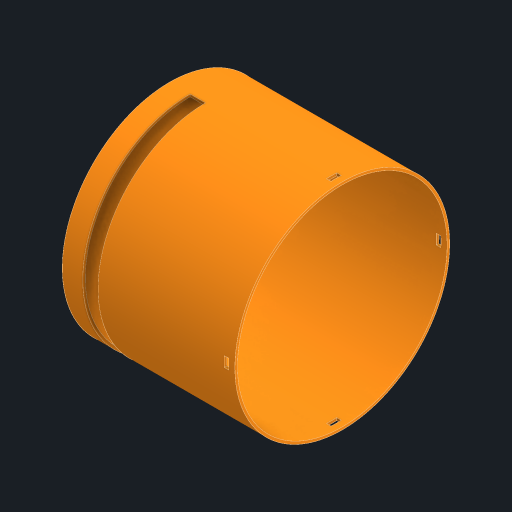
# Autodesk Inventor part: OUTK_001_ChipBucket
Saved by Autodesk Inventor 2024.2 (Build 282272000, 272)
## iProperties
Created: 2024-11-24
Part Number: OUTK_001_ChipBucket
Material: Polyethylene, High Density
Document SubType Name: Modeling
Designer: Bryan
Density: 0.952 g/cm^3
Appearance: Orange
Mass: 1203.08 g
Surface Area: 4862.89 cm^2
Volume: 1263.74 cm^3
Author: Bryan
Autodesk Inventor part; units mm, degrees
ref_plane "YZ Plane" through (0, 0, 0) normal (1, 0, 0) x (0, 1, 0)
ref_plane "XZ Plane" through (0, 0, 0) normal (0, 1, 0) x (-1, 0, 0)
ref_plane "XY Plane" through (0, 0, 0) normal (0, 0, 1) x (1, 0, 0)
sketch "Sketch1" plane through (0, 0, 0) normal (1, 0, 0) x (0, 1, 0)
  circle A0 centre (0, 0) radius 133.35
  dimension "d0" = 266.7
  constraints: 1 centre point, 1 coincident
  measures "d0" diameter of A0
extrude "Extrusion1" add sketch "Sketch1" along normal mid plane 214.3435
sketch "Sketch2" plane through (107.1717, 0, 0) normal (1, 0, 0) x (0, 0, -1)
  circle A0 centre (0, 0) radius 130.175
  dimension "d3" = 260.35
  constraints: 1 centre point, 1 coincident
  measures "d3" diameter of A0
extrude "Extrusion2" cut sketch "Sketch2" against normal blind 201.6435
sketch "Sketch3" plane through (0, 0, 0) normal (0, 0, 1) x (1, 0, 0)
  line L0 (107.1717, 130.175) -> (107.1717, -130.175) projected
  line L1 (107.1717, 130.175) -> (-94.4717, 130.175) projected
  line L2 (107.1717, -130.175) -> (-94.4717, -130.175) projected
  line L3 (-81.7717, 130.175) -> (-81.7717, -130.175)
  line L4 (-62.7217, -130.175) -> (-62.7217, 130.175)
  line L5 (-94.4717, 130.175) -> (-94.4717, -130.175) projected
  point P0 (0, 0)
  point P1 (-139.7, 130.175)
  point P2 (-139.7, -130.175)
  dimension "d7" = 19.05
  dimension "d61" = 12.7
  constraints: 4 end point, 4 point on line, 1 parallel, 1 vertical
  measures "d7" distance between parallel lines of L3 L4
  measures "d61" distance between parallel lines of L3 L5
extrude "Extrusion3" cut sketch "Sketch3" along normal blind 266.7 contours L4 L2 L3 L1
sketch "Sketch4" plane through (0, 0, 0) normal (0, 1, 0) x (-1, 0, 0)
  line L0 (81.7717, 0) -> (62.7217, 0) projected
  line L1 (81.7717, 0) -> (81.7717, 28.9256) projected
  line L2 (62.7217, 0) -> (62.7217, 28.9256) projected
  line L3 (62.7217, 28.9256) -> (81.7717, 28.9256) projected
  point P0 (0, 0)
extrude "Extrusion4" cut sketch "Sketch4" along normal through all both and the other way through all
sketch "Sketch5" plane through (0, 0, 0) normal (0, 1, 0) x (-1, 0, 0)
  line L0 (-93.8367, 6.35) -> (-99.5517, 6.35)
  line L1 (-99.5517, 6.35) -> (-99.5517, -6.35)
  line L2 (-99.5517, -6.35) -> (-93.8367, -6.35)
  line L3 (-93.8367, -6.35) -> (-93.8367, 6.35)
  line L4 (-107.1717, 133.35) -> (-107.1717, -133.35) projected
  point P0 (0, 0)
  point P1 (-93.8367, 0)
  dimension "d12" = 5.715
  dimension "d13" = 12.7
  dimension "d14" = 7.62
  constraints: 8 end point, 2 parallel, 1 horizontal, 1 horizontal alignment, 1 midpoint, 1 perpendicular
  measures "d12" distance of L2.end L1.end
  measures "d13" distance of L1.end L0.end
  measures "d14" distance between parallel lines of L4 L1
extrude "Extrusion5" cut sketch "Sketch5" along normal through all both and the other way through all
sketch "Sketch6" plane through (0, 0, 0) normal (0, 0, 1) x (1, 0, 0)
  line L0 (93.8367, 6.35) -> (99.5517, 6.35)
  line L1 (99.5517, 6.35) -> (99.5517, -6.35)
  line L2 (99.5517, -6.35) -> (93.8367, -6.35)
  line L3 (93.8367, -6.35) -> (93.8367, 6.35)
  line L4 (107.1717, -133.35) -> (107.1717, 133.35) projected
  point P0 (0, 0)
  point P1 (93.8367, 0)
  dimension "d17" = 5.715
  dimension "d18" = 12.7
  dimension "d19" = 7.62
  constraints: 8 end point, 2 parallel, 1 horizontal, 1 horizontal alignment, 1 midpoint, 1 perpendicular
  measures "d17" distance of L1.end L2.end
  measures "d18" distance of L0.end L1.end
  measures "d19" distance between parallel lines of L4 L1
extrude "Extrusion6" cut sketch "Sketch6" along normal through all both and the other way through all
sketch "Sketch8" plane through (-107.1717, 0, 0) normal (-1, 0, 0) x (0, 0, 1)
  line L0 (10.1087, 20) -> (-10.1087, 20)
  arc A0 (10.5941, 19.6202) -> (10.1087, 20) centre (10.1087, 19.5) ccw
  line L1 (12.6118, 11.4728) -> (10.5941, 19.6202)
  arc A1 (12.6118, 11.4728) -> (13.7322, 10.7244) centre (13.5825, 11.7132) ccw
  arc A2 (15.3907, 3.9529) -> (13.7322, 10.7244) centre (14.2561, 7.2639) ccw
  arc A3 (15.3907, 3.9529) -> (14.7327, 2.8189) centre (15.7149, 3.0069) ccw
  arc A4 (13.721, -6.0608) -> (14.7327, 2.8189) centre (0, 0) ccw
  arc A5 (13.721, -6.0608) -> (14.1071, -7.3137) centre (14.6358, -6.4649) ccw
  arc A6 (9.6523, -12.6228) -> (14.1071, -7.3137) centre (12.2567, -10.2846) ccw
  line L2 (-10.5941, 19.6202) -> (-12.6118, 11.4728)
  arc A7 (-10.1087, 20) -> (-10.5941, 19.6202) centre (-10.1087, 19.5) ccw
  arc A8 (-13.7322, 10.7244) -> (-12.6118, 11.4728) centre (-13.5825, 11.7132) ccw
  arc A9 (-13.7322, 10.7244) -> (-15.3907, 3.9529) centre (-14.2561, 7.2639) ccw
  arc A10 (-14.7327, 2.8189) -> (-15.3907, 3.9529) centre (-15.7149, 3.0069) ccw
  arc A11 (-14.7327, 2.8189) -> (-13.721, -6.0608) centre (0, 0) ccw
  arc A12 (-14.1071, -7.3137) -> (-13.721, -6.0608) centre (-14.6358, -6.4649) ccw
  arc A13 (-14.1071, -7.3137) -> (-9.6523, -12.6228) centre (-12.2567, -10.2846) ccw
  arc A14 (-8.3514, -12.4601) -> (-9.6523, -12.6228) centre (-8.9081, -13.2908) ccw
  arc A15 (-8.3514, -12.4601) -> (8.3514, -12.4601) centre (0, 0) ccw
  arc A16 (9.6523, -12.6228) -> (8.3514, -12.4601) centre (8.9081, -13.2908) ccw
  circle A17 centre (0, -36.5002) radius 19.8
  circle A18 centre (0, -36.5002) radius 6.5
  line L3 (0, 20) -> (0, -15) construction
  line L4 (-12.2567, -10.2846) -> (-12.2567, 7.2639) construction
  line L5 (-12.2567, 7.2639) -> (-14.2561, 7.2639) construction
  line L6 (-14.2561, 7.2639) -> (-12.2567, -10.2846) construction
  line L7 (-12.2567, -10.2846) -> (12.2567, -10.2846) construction
  line L8 (-14.2561, 7.2639) -> (14.2561, 7.2639) construction
  circle A19 centre (-26.9875, 23.175) radius 3.2512
  circle A20 centre (-26.9875, -6.6626) radius 3.2512
  circle A21 centre (26.9875, 23.175) radius 3.2512
  circle A22 centre (26.9875, -6.6626) radius 3.2512
  circle A23 centre (-26.9875, -36.5002) radius 3.2512
  circle A24 centre (26.9875, -36.5002) radius 3.2512
  line L9 (-26.9875, 23.175) -> (-26.9875, -6.6626) construction
  line L10 (-26.9875, -6.6626) -> (-26.9875, -36.5002) construction
  line L11 (-26.9875, -36.5002) -> (26.9875, -36.5002) construction
  line L12 (26.9875, -36.5002) -> (26.9875, -6.6626) construction
  line L13 (26.9875, -6.6626) -> (26.9875, 23.175) construction
  line L14 (26.9875, 23.175) -> (-26.9875, 23.175) construction
  point P0 (0, 23.175)
  point P1 (0, -36.5002)
  dimension "d66" = 20.2174
  dimension "d67" = 0.5
  dimension "d68" = 3.5
  dimension "d69" = 1
  dimension "d70" = 15
  dimension "d71" = 8.3935
  dimension "d72" = 103.91
  dimension "d73" = 83.5
  dimension "d74" = 20
  dimension "d75" = 17.5485
  dimension "d76" = 24.5134
  dimension "d77" = 28.5121
  dimension "d78" = 13
  dimension "d79" = 39.6
  dimension "d80" = 36.5002
  dimension "d81" = 6.5024
  dimension "d82" = 3.175
  dimension "d83" = 53.975
  dimension "d84" = 29.845
  constraints: 35 point on circle, 30 end point, 25 centre point, 19 tangent, 18 equal radius, 6 vertical alignment, 5 coincident, 5 horizontal, 5 horizontal alignment, 5 vertical, 3 midpoint, 2 equal length, 2 perpendicular, 1 point on line, 1 other
  measures "d66" distance of L0.start L0.end
  measures "d67" radius of A7
  measures "d68" radius of A9
  measures "d69" radius of A8
  measures "d70" radius of A11
  measures "d71" distance of L2.start L2.end
  measures "d72" angle of L0 L2
  measures "d73" angle of L5 L6
  measures "d74" distance from line of L0 A4.centre
  measures "d75" vertical distance of L5.end L4.start
  measures "d76" distance of L7.end L4.start
  measures "d77" distance of L5.end L8.end
  measures "d78" diameter of A18
  measures "d79" diameter of A17
  measures "d80" distance of A4.centre A17.centre
  measures "d81" diameter of A19
  measures "d82" distance between parallel lines of L0 L14
  measures "d83" distance of L13.end L9.start
extrude "Extrusion7" [suppressed]
sketch "Sketch10" plane through (-107.1717, 0, 0) normal (-1, 0, 0) x (0, 0, 1)
  circle A0 centre (9.7202, -76.2) radius 2.54
  circle A1 centre (9.7202, -123.1331) radius 2.54
  circle A2 centre (-9.7202, -76.2) radius 2.54
  circle A3 centre (-9.7202, -123.1331) radius 2.54
  line L0 (0, 186.69) -> (0, -186.69) projected
  line L1 (-9.525, -50.8) -> (-9.525, 50.8) projected
  line L2 (-9.525, 50.8) -> (9.525, 50.8) projected
  line L3 (9.525, -50.8) -> (-9.525, -50.8) projected
  line L4 (-9.7202, -76.2) -> (9.7202, -123.1331) construction
  line L5 (-9.7202, -123.1331) -> (9.7202, -76.2) construction
  circle A4 centre (0, -99.6665) radius 9.525
  circle A5 centre (0, -99.6665) radius 25.4
  dimension "d100" = 50.8
  dimension "d89" = 5.08
  dimension "d91" = 19.4403
  dimension "d98" = 25.4
  dimension "d99" = 19.05
  constraints: 5 centre point, 4 end point, 3 equal radius, 2 horizontal alignment, 2 vertical alignment, 1 coincident, 1 midpoint, 1 symmetric about line, 3 other
  measures "d89" diameter of A2
  measures "d91" distance of L5.end L4.start
  measures "d98" distance from line of L3 L5.end
  measures "d99" diameter of A4
extrude "Extrusion9" cut sketch "Sketch10" against normal blind 201.6435 contours A0 A5 | A5 A0 | A5 A2 | A2 A5 | A5 A1 | A1 A5 | A5 A3 | A3 A5
body "Solid1"
